Autodesk Inventor part; units mm, degrees
(part 3 of 3)
  spline S466 degree 2 poles (172.2072, -108.4164) (172.1831, -108.5) (172.0899, -108.5) knots 0 0 0 1 1 1
  spline S467 degree 2 poles (174.3878, -108.0484) (174.3878, -108.1609) (174.2673, -108.1609) knots 0 0 0 1 1 1
  spline S468 degree 2 poles (174.2673, -108.1609) (174.1789, -108.1609) (174.1516, -108.0854) knots 0 0 0 1 1 1
  line L304 (174.1516, -108.0854) -> (174.023, -107.7367)
  line L305 (174.023, -107.7367) -> (173.3883, -107.7367)
  line L306 (173.3883, -107.7367) -> (173.2613, -108.0854)
  spline S469 degree 2 poles (173.2613, -108.0854) (173.234, -108.1609) (173.1456, -108.1609) knots 0 0 0 1 1 1
  spline S470 degree 2 poles (173.1456, -108.1609) (173.0251, -108.1609) (173.0251, -108.0484) knots 0 0 0 1 1 1
  spline S471 degree 2 poles (173.0251, -108.0484) (173.0251, -108.0275) (173.0315, -108.0131) knots 0 0 0 1 1 1
  line L307 (173.0315, -108.0131) -> (173.586, -106.5315)
  spline S472 degree 2 poles (173.586, -106.5315) (173.6197, -106.4109) (173.7065, -106.4109) knots 0 0 0 1 1 1
  spline S473 degree 2 poles (173.7065, -106.4109) (173.7933, -106.4109) (173.8238, -106.4929) knots 0 0 0 1 1 1
  line L308 (173.8238, -106.4929) -> (174.3814, -108.0131)
  spline S474 degree 2 poles (174.3814, -108.0131) (174.3878, -108.0292) (174.3878, -108.0484) knots 0 0 0 1 1 1
  spline S475 degree 2 poles (173.8929, -106.1233) (173.8254, -106.1233) (173.7579, -106.0895) knots 0 0 0 1 1 1
  spline S476 degree 2 poles (173.7579, -106.0895) (173.6888, -106.0494) (173.6518, -106.0285) knots 0 0 0 1 1 1
  spline S477 degree 2 poles (173.6518, -106.0285) (173.6229, -106.0172) (173.5699, -105.9787) knots 0 0 0 1 1 1
  spline S478 degree 2 poles (173.5699, -105.9787) (173.5361, -105.9545) (173.5201, -105.9545) knots 0 0 0 1 1 1
  spline S479 degree 2 poles (173.5201, -105.9545) (173.4911, -105.9545) (173.3803, -106.0381) (173.3337, -106.0381) knots 0 0 0 1 2 2 2
  spline S480 degree 2 poles (173.3337, -106.0381) (173.2854, -106.0381) (173.2115, -105.9722) (173.2115, -105.9272) knots 0 0 0 1 2 2 2
  spline S481 degree 2 poles (173.2115, -105.9272) (173.2115, -105.871) (173.3047, -105.8308) knots 0 0 0 1 1 1
  spline S482 degree 2 poles (173.3047, -105.8308) (173.3529, -105.7762) (173.3899, -105.7585) knots 0 0 0 1 1 1
  spline S483 degree 2 poles (173.3899, -105.7585) (173.4429, -105.7312) (173.5201, -105.7312) knots 0 0 0 1 1 1
  spline S484 degree 2 poles (173.5201, -105.7312) (173.5811, -105.7312) (173.6518, -105.7649) knots 0 0 0 1 1 1
  spline S485 degree 2 poles (173.6518, -105.7649) (173.7017, -105.7922) (173.7499, -105.8196) knots 0 0 0 1 1 1
  spline S486 degree 2 poles (173.7499, -105.8196) (173.782, -105.8324) (173.8399, -105.8742) knots 0 0 0 1 1 1
  spline S487 degree 2 poles (173.8399, -105.8742) (173.8768, -105.9015) (173.8929, -105.9015) knots 0 0 0 1 1 1
  spline S488 degree 2 poles (173.8929, -105.9015) (173.9218, -105.9015) (174.0343, -105.8163) (174.0793, -105.8163) knots 0 0 0 1 2 2 2
  spline S489 degree 2 poles (174.0793, -105.8163) (174.1998, -105.8163) (174.1998, -105.9272) knots 0 0 0 1 1 1
  spline S490 degree 2 poles (174.1998, -105.9272) (174.1998, -105.9787) (174.15, -106.0188) knots 0 0 0 1 1 1
  spline S491 degree 2 poles (174.15, -106.0188) (174.113, -106.0429) (174.0761, -106.0686) knots 0 0 0 1 1 1
  spline S492 degree 2 poles (174.0761, -106.0686) (173.9941, -106.1233) (173.8929, -106.1233) knots 0 0 0 1 1 1
  line L309 (173.7065, -106.8175) -> (173.459, -107.5133)
  line L310 (173.459, -107.5133) -> (173.9539, -107.5133)
  line L311 (173.9539, -107.5133) -> (173.7065, -106.8175)
  spline S493 degree 2 poles (175.9177, -107.6242) (175.9177, -107.8476) (175.5722, -108.1609) (175.3295, -108.1609) knots 0 0 0 1 2 2 2
  spline S494 degree 2 poles (175.3295, -108.1609) (175.0853, -108.1609) (174.7414, -107.8476) (174.7414, -107.6242) knots 0 0 0 1 2 2 2
  line L312 (174.7414, -107.6242) -> (174.7414, -106.9444)
  spline S495 degree 2 poles (174.7414, -106.9444) (174.7414, -106.7227) (175.0853, -106.4093) (175.3295, -106.4093) knots 0 0 0 1 2 2 2
  spline S496 degree 2 poles (175.3295, -106.4093) (175.5738, -106.4093) (175.9177, -106.7211) (175.9177, -106.9444) knots 0 0 0 1 2 2 2
  line L313 (175.9177, -106.9444) -> (175.9177, -107.6242)
  line L314 (175.6766, -107.6242) -> (175.6766, -106.9444)
  spline S497 degree 2 poles (175.6766, -106.9444) (175.6766, -106.8143) (175.4758, -106.6327) (175.3295, -106.6327) knots 0 0 0 1 2 2 2
  spline S498 degree 2 poles (175.3295, -106.6327) (175.1833, -106.6327) (174.9824, -106.8143) (174.9824, -106.9444) knots 0 0 0 1 2 2 2
  line L315 (174.9824, -106.9444) -> (174.9824, -107.6242)
  spline S499 degree 2 poles (174.9824, -107.6242) (174.9824, -107.756) (175.1833, -107.9376) (175.3295, -107.9376) knots 0 0 0 1 2 2 2
  spline S500 degree 2 poles (175.3295, -107.9376) (175.4758, -107.9376) (175.6766, -107.756) (175.6766, -107.6242) knots 0 0 0 1 2 2 2
  point P0 (0, 0)
  point P1 (-185.4, -105)
  point P2 (142.4, -101.5)
  point P3 (145.4, -105)
  point P4 (181.9, -106.5)
  point P5 (185.4, -105)
  dimension "d224" = 4
  dimension "d225" = 5
  dimension "d241" = 33
  dimension "d242" = 40
  dimension "d243" = 4
  dimension "d244" = 7
  dimension "d245" = 3
  dimension "d246" = 1.5
  constraints: 6 midpoint, 2 collinear, 2 end point, 2 horizontal, 1 parallel, 1 perpendicular, 1 point on line, 8 other
  measures "d224" distance between parallel lines of L3 L1
  measures "d225" distance from line of L4 point (-185.4, -105)
  measures "d241" distance from line of point (181.9, -106.5) L7
  measures "d242" distance from line of point (185.4, -105) L6
  measures "d243" distance between parallel lines of L12 L10
  measures "d244" distance between parallel lines of L12 L14
  measures "d245" distance from line of L6 point (142.4, -101.5)
  measures "d246" distance from line of L4 L6.start
emboss "Relevo1" sketch "Esboço27" operation cut depth 0.1 direction (0, 0, -1)
